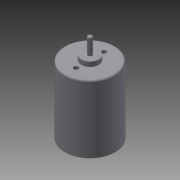
# Autodesk Inventor part: Nidec_DMN29
Saved by Autodesk Inventor 2016 (Build 200138000, 138)
## iProperties
Created: 2016-01-21
Part Number: Nidec_DMN29
Material: Générique
Document SubType Name: Modeling
Designer: sd
Density: 3.45016 g/cm^3
Appearance: Par défaut
Mass: 90 g
Surface Area: 51.2202 cm^2
Volume: 26.0857 cm^3
Author: sd
Autodesk Inventor part; units mm, degrees
ref_plane "YZ Plane" through (0, 0, 0) normal (1, 0, 0) x (0, 1, 0)
ref_plane "XZ Plane" through (0, 0, 0) normal (0, 1, 0) x (-1, 0, 0)
ref_plane "XY Plane" through (0, 0, 0) normal (0, 0, 1) x (1, 0, 0)
sketch "Esquisse1" plane through (0, 0, 0) normal (0, 0, 1) x (1, 0, 0)
  circle A0 centre (0, 0) radius 14.5
  dimension "d0" = 29
  constraints: 1 centre point, 1 coincident
  measures "d0" diameter of A0
extrude "Extrusion1" add sketch "Esquisse1" along normal blind 38.8
sketch "Esquisse2" plane through (0, 0, 38.8) normal (0, 0, 1) x (1, 0, 0)
  circle A0 centre (0, 0) radius 14.5 projected
  circle A1 centre (0, 0) radius 5
  dimension "d3" = 10
  constraints: 1 centre point, 1 coincident
  measures "d3" diameter of A1
extrude "Extrusion2" add sketch "Esquisse2" along normal blind 2.7 contours A1
sketch "Esquisse3" plane through (0, 0, 41.5) normal (0, 0, 1) x (1, 0, 0)
  circle A0 centre (0, 0) radius 5 projected
  circle A1 centre (0, 0) radius 1.25
  dimension "d6" = 2.5
  constraints: 1 centre point, 1 coincident
  measures "d6" diameter of A1
extrude "Extrusion3" add sketch "Esquisse3" along normal blind 9.3 contours A1
sketch "Esquisse4" plane through (0, 0, 0) normal (0, 0, -1) x (-1, 0, 0)
  circle A0 centre (0, 0) radius 14.5 projected
  circle A1 centre (0, 0) radius 5
  dimension "d9" = 10
  constraints: 1 centre point, 1 coincident
  measures "d9" diameter of A1
extrude "Extrusion4" add sketch "Esquisse4" along normal blind 3.2 contours A1
fillet "Congé1" radius 1 1 edges at (-14.5, 0, 38.8)
fillet "Congé2" radius 0.5 1 edges at (-1.25, 0, 50.8)
sketch "Esquisse5" plane through (0, 0, 38.8) normal (0, 0, 1) x (1, 0, 0)
  circle A0 centre (0, 0) radius 5 projected
  circle A1 centre (0, 8) radius 1.3
  circle A2 centre (0, -8) radius 1.3
  dimension "d14" = 2.6
  dimension "d15" = 8
  dimension "d16" = 2.6
  dimension "d17" = 8
  constraints: 2 centre point
  measures "d14" diameter of A1
  measures "d15" distance of A0.centre A1.centre
  measures "d16" diameter of A2
  measures "d17" distance of A0.centre A2.centre
extrude "Extrusion5" cut sketch "Esquisse5" against normal blind 3 contours A1 | A2
thread "Filetage1" size "M3x0.5" class "6H" standard "ANSI Metric M Profile" full length
thread "Filetage2" size "M3x0.5" class "6H" standard "ANSI Metric M Profile" full length
equation "\"d16\" = d14"
equation "\"d17\" = d15"
